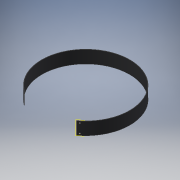
# Autodesk Inventor part: 3rdShroud
Saved by Autodesk Inventor 2017 (Build 210142000, 142)
## iProperties
Created: 2019-07-01
Part Number: 3rdShroud
Material: Generic
Document SubType Name: Modeling
Designer: cresswnd
Density: 1 g/cm^3
Appearance: Generic
Author: cresswnd
Autodesk Inventor part; units mm, degrees
ref_plane "YZ Plane" through (0, 0, 0) normal (1, 0, 0) x (0, 1, 0)
ref_plane "XZ Plane" through (0, 0, 0) normal (0, 1, 0) x (-1, 0, 0)
ref_plane "XY Plane" through (0, 0, 0) normal (0, 0, 1) x (1, 0, 0)
sketch "Sketch1" plane through (0, 0, 0) normal (0, 0, 1) x (1, 0, 0)
  arc A0 (62.3383, -89.7392) -> (-62.3386, -89.7387) centre (0.0001, -5.2464) ccw
  arc A1 (61.8662, -89.0928) -> (-61.866, -89.0928) centre (0.0001, -5.2464) ccw
  line L0 (-62.3386, -89.7387) -> (-61.866, -89.0928)
  line L1 (62.3383, -89.7392) -> (61.8662, -89.0928)
  point P0 (0, 0)
  dimension "d0" = 208.4
  constraints: 4 end point, 4 point on circle, 2 centre point, 1 coincident
  measures "d0" diameter of A1
extrude "Extrusion1" add sketch "Sketch1" along normal blind 30
ref_plane "Work Plane1" through (61.0727, -89.6701, 0) normal (0.6382, -0.7699, 0) x (0.7699, 0.6382, 0)
sketch "Sketch2" plane through (61.0727, -89.6701, 0) normal (0.6382, -0.7699, 0) x (0.7699, 0.6382, 0)
  circle A0 centre (6.5, 25.5) radius 1.4 projected
  circle A1 centre (6.5, 4.5) radius 1.4 projected
  point P0 (10.2035, 0)
extrude "Extrusion2" cut sketch "Sketch2" along normal blind 30
mirror "Mirror1" about plane through (0, 0, 0) normal (1, 0, 0) of "Extrusion2"
body "Solid1"
